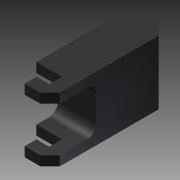
# Autodesk Inventor part: D-044
Saved by Autodesk Inventor 2015 (Build 190159000, 159)
## iProperties
Company: MARCHA TECHNOLOGY
Created: 2013-10-23
Part Number: D-044
Document SubType Name: Modeling
Designer: O.Martin
Density: 1 g/cm^3
Project: WITBOXprinter_K01
Description: SOPORTE  POLEA LIBRE
Stock Number: 28655
Material: Generic
Appearance: Rubber - Black - Version 1.1
Author: O.Martin
Autodesk Inventor part; units mm, degrees
ref_plane "YZ Plane" through (0, 0, 0) normal (1, 0, 0) x (0, 1, 0)
ref_plane "XZ Plane" through (0, 0, 0) normal (0, 1, 0) x (-1, 0, 0)
ref_plane "XY Plane" through (0, 0, 0) normal (0, 0, 1) x (1, 0, 0)
sketch "Boceto1" plane through (0, 0, 0) normal (0, 0, 1) x (1, 0, 0)
  line L0 (-1.3279, 11.1925) -> (10.6721, 11.1925)
  line L1 (10.6721, 11.1925) -> (10.6721, -25.8075)
  line L2 (10.6721, -25.8075) -> (-1.3279, -25.8075)
  line L3 (-1.3279, -25.8075) -> (-1.3279, 11.1925)
  line L4 (-1.3279, -18.1075) -> (6.6721, -18.1075)
  line L5 (6.6721, -18.1075) -> (6.6721, -22.1075)
  line L6 (6.6721, -22.1075) -> (-1.3279, -22.1075)
  line L7 (-1.3279, -22.1075) -> (-1.3279, -18.1075)
  line L8 (6.6721, -20.1075) -> (-1.3279, -20.1075) construction
  line L9 (2.6721, -22.1075) -> (2.6721, -25.8075)
  dimension "d0" = 12
  dimension "d1" = 37
  dimension "d2" = 31.3
  dimension "d3" = 4
  dimension "d4" = 4
  dimension "d25" = 8
  constraints: 20 end point, 4 parallel, 3 midpoint, 3 perpendicular, 2 horizontal, 2 point on line
  measures "d0" distance of L0.start L0.end
  measures "d1" distance of L0.end L1.end
  measures "d2" distance between parallel lines of L0 L8
  measures "d3" distance of L4.end L5.end
  measures "d4" distance between parallel lines of L5 L9
  measures "d25" distance of L4.start L4.end
extrude "Extrusión1" add sketch "Boceto1" along normal mid plane 20 contours L0 L1 L2 L9 L6 L5 L4 L3
sketch "Boceto2" plane through (-1.3279, -18.1075, 10) normal (-1, 0, 0) x (0, 0, 1)
  line L0 (0, 29.3) -> (-20, 29.3) projected
  line L1 (-20, 0) -> (0, 0) projected
  line L2 (-10, 24.3) -> (-10, 11.8) construction
  point P0 (-10, 29.3)
  dimension "d8" = 12.5
  dimension "d9" = 5
  constraints: 2 coincident, 2 end point, 1 midpoint, 1 perpendicular, 1 vertical alignment
  measures "d8" distance of L2.start L2.end
  measures "d9" distance from line of L0 L2.start
hole "Agujero1" at (-1.3279, 6.1925, 0) at (-1.3279, -6.3075, 0) direction (1, 0, 0) diameter 3.242 depth 8 tip angle 118 thread size "M4x0.7" class "6H" standard "ISO Metric profile"
sketch "Boceto3" plane through (10.6721, -25.8075, 10) normal (1, 0, 0) x (0, 0, -1)
  line L0 (20, 37) -> (0, 37) projected
  line L1 (20, 0) -> (0, 0) projected
  line L2 (3, 0) -> (17, 0)
  line L3 (17, 0) -> (17, 14.5)
  line L4 (17, 14.5) -> (3, 14.5)
  line L5 (3, 14.5) -> (3, 0)
  point P0 (10, 14.5)
  point P1 (10, 37)
  dimension "d17" = 22.5
  dimension "d18" = 14
  constraints: 8 end point, 2 midpoint, 2 parallel, 1 horizontal, 1 perpendicular, 1 point on line, 1 vertical alignment
  measures "d17" distance between parallel lines of L0 L4
  measures "d18" distance of L3.end L4.end
extrude "Extrusión2" cut sketch "Boceto3" against normal through all
fillet "Empalme1" radius 3 2 edges at (4.6721, -11.3075, 7) (4.6721, -11.3075, -7)
chamfer "Chaflán1" distance 3 angle 45 3 edges at (10.6721, 11.1925, 0) (10.6721, -25.8075, 8.5) (10.6721, -25.8075, -8.5)
body "Solid1"
